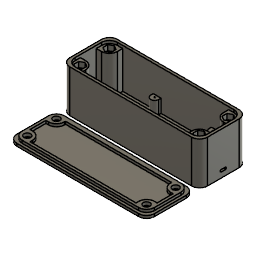
RGB Box v1 (Autodesk Fusion 360 design; units mm, degrees)
Autodesk Fusion 360 part; units mm, degrees
sketch "Sketch1" plane through (0, 0, 0) normal (0, 1, 0) x (1, 0, 0)
  line L0 (0, 0) -> (127, 0)
  line L1 (127, 0) -> (127, 40.64)
  line L2 (127, 40.64) -> (0, 40.64)
  line L3 (0, 40.64) -> (0, 0)
  line L4 (-2.54, -2.54) -> (129.54, -2.54)
  line L5 (129.54, -2.54) -> (129.54, 43.18)
  line L6 (129.54, 43.18) -> (-2.54, 43.18)
  line L7 (-2.54, 43.18) -> (-2.54, -2.54)
  line L8 (129.54, -2.54) -> (110.49, -2.54)
  line L9 (110.49, -2.54) -> (110.49, 16.51)
  line L10 (110.49, 16.51) -> (129.54, 16.51)
  line L11 (129.54, 16.51) -> (129.54, -2.54)
  line L12 (129.54, 43.18) -> (110.49, 43.18)
  line L13 (110.49, 43.18) -> (110.49, 24.13)
  line L14 (110.49, 24.13) -> (129.54, 24.13)
  line L15 (129.54, 24.13) -> (129.54, 43.18)
  dimension "d1" = 127
  dimension "d2" = 40.64
  dimension "d3" = 2.54
  dimension "d45" = 19.05
  dimension "d46" = 19.05
  dimension "d47" = 19.05
  dimension "d48" = 19.05
  constraint horizontal L0
  constraint vertical L1
  constraint horizontal L2
  constraint vertical L3
  constraint coincident L0.start L3.end
  constraint horizontal L8
  constraint vertical L9
  constraint horizontal L10
  constraint vertical L11
  constraint horizontal L12
  constraint vertical L13
  constraint horizontal L14
  constraint vertical L15
  measures "d1" distance of L0.start L0.end
  measures "d2" distance of L0.start L2.end
  measures "d45" distance of L4.end L8.end
  measures "d46" distance of L4.end L10.end
  measures "d47" distance of L5.end L12.end
  measures "d48" distance of L5.end L14.end
extrude "Extrude1" add sketch "Sketch1" along normal blind 40.64 makes body 1
shell "Shell1" thickness 2.54 removed faces 1 at (72.8133, 40.64, -12.7) on bodies 1
fillet "Fillet1" radius 7.62 8 edges at (0, 21.59, -40.64) (-2.54, 20.32, -43.18) (0, 21.59, 0) (-2.54, 20.32, 2.54) (127, 21.59, -40.64) (129.54, 20.32, -43.18) (127, 21.59, 0) (129.54, 20.32, 2.54) on bodies 1
sketch "Sketch2" plane through (-2.54, 0, 0) normal (-1, 0, 0) x (0, 0, 1)
  line L0 (-5.08, 0) -> (-5.08, 40.64)
  line L1 (-5.08, 40.64) -> (-35.56, 40.64)
  line L2 (-35.56, 40.64) -> (-35.56, 0)
  line L3 (-35.56, 0) -> (-5.08, 0)
  line L4 (-20.32, 0) -> (-20.32, 2.54)
  line L5 (-20.32, 2.54) -> (-20.32, 3.429)
  circle A0 centre (-20.32, 8.3185) radius 4.8895
  circle A1 centre (-20.32, 8.3185) radius 3.4925
  line L6 (-25.2095, 8.3185) -> (-15.4305, 8.3185)
  line L7 (-15.4305, 8.3185) -> (-15.4305, 0)
  line L8 (-15.4305, 0) -> (-25.2095, 0)
  line L9 (-25.2095, 0) -> (-25.2095, 8.3185)
  line L10 (-15.4305, 0) -> (-14.1605, 0)
  line L11 (-14.1605, 0) -> (-14.1605, 8.3172)
  line L12 (-14.1605, 8.3172) -> (-15.4305, 8.3172)
  line L13 (-15.4305, 8.3172) -> (-15.4305, 0)
  line L14 (-25.2095, 8.3185) -> (-26.4795, 8.3185)
  line L15 (-26.4795, 8.3185) -> (-26.4795, 0)
  line L16 (-26.4795, 0) -> (-25.2095, 0)
  line L17 (-25.2095, 0) -> (-25.2095, 8.3185)
  dimension "d9" = 0.889
  dimension "d10" = 9.779
  dimension "d11" = 6.985
  dimension "d12" = 9.779
  dimension "d16" = 1.27
  dimension "d17" = 1.27
  constraint midpoint L3 L4.start
  constraint perpendicular L3 L4
  constraint perpendicular L3 L5
  constraint coincident L5.end A0
  constraint concentric A0 A1
  constraint horizontal L6
  constraint vertical L7
  constraint horizontal L8
  constraint vertical L9
  constraint coincident L3 L7.end
  constraint coincident A0 L6.start
  constraint horizontal L10
  constraint vertical L11
  constraint horizontal L12
  constraint vertical L13
  constraint horizontal L14
  constraint vertical L15
  constraint horizontal L16
  constraint vertical L17
  constraint coincident L3 L15.end
  measures "d9" distance of L4.end L5.end
  measures "d10" diameter of A0
  measures "d11" diameter of A1
  measures "d12" distance of L6.start L6.end
  measures "d16" distance of L7.end L10.end
  measures "d17" distance of L6.start L14.end
extrude "Extrude2" add sketch "Sketch2" against normal blind 8.89 from surface at -2.54 contours L3 L7 L10 L11 L12 L13 | L3 L4 L5 A0 L7 L8 L13 | L3 L4 L5 A0 L8 L9 L17 | L3 L9 L14 L15 L16 L17 bodies 1
extrude "Extrude3" cut sketch "Sketch2" against normal blind 8.89 contours A1 L6 | A1 L6 bodies 1
sketch "Sketch3" plane through (0, 2.54, 0) normal (0, 1, 0) x (-1, 0, 0)
  line L0 (-8.89, -14.1605) -> (0, -14.1605)
  line L1 (0, -14.1605) -> (0, -7.62)
  arc A0 (0, -7.62) -> (-7.62, 0) centre (-7.62, -7.62) ccw
  line L2 (-7.62, 0) -> (-119.38, 0)
  arc A1 (-119.38, 0) -> (-127, -7.62) centre (-119.38, -7.62) ccw
  line L3 (-127, -7.62) -> (-127, -33.02)
  arc A2 (-127, -33.02) -> (-119.38, -40.64) centre (-119.38, -33.02) ccw
  line L4 (-119.38, -40.64) -> (-7.62, -40.64)
  arc A3 (-7.62, -40.64) -> (0, -33.02) centre (-7.62, -33.02) ccw
  line L5 (0, -33.02) -> (0, -26.4795)
  line L6 (0, -26.4795) -> (-8.89, -26.4795)
  line L7 (-8.89, -26.4795) -> (-8.89, -14.1605)
  line L8 (0, -14.1605) -> (-33.528, -14.1605)
  line L9 (-33.528, -14.1605) -> (-33.528, -26.4795)
  line L10 (-33.528, -26.4795) -> (-37.846, -26.4795)
  line L11 (-37.846, -26.4795) -> (-37.846, -14.1605)
  line L12 (-37.846, -14.1605) -> (-33.528, -14.1605)
  line L13 (-33.528, -14.1605) -> (-33.528, -26.4795)
  dimension "d20" = 33.528
  dimension "d21" = 4.318
  constraint coincident L0.end L1.start
  constraint perpendicular L1 L8
  constraint perpendicular L6 L9
  constraint horizontal L10
  constraint vertical L11
  constraint horizontal L12
  constraint vertical L13
  measures "d20" distance of L0.end L8.end
  measures "d21" distance of L9.end L10.end
extrude "Extrude4" add sketch "Sketch3" along normal blind 1.905 contours L9 L10 L11 L12 L13 bodies 1
sketch "Sketch4" plane through (129.54, 0, 0) normal (1, 0, 0) x (0, 0, -1)
  line L0 (5.08, 40.64) -> (5.08, 0)
  line L1 (5.08, 0) -> (35.56, 0)
  line L2 (35.56, 0) -> (35.56, 40.64)
  line L3 (35.56, 40.64) -> (5.08, 40.64)
  line L4 (20.32, 0) -> (20.32, 2.54)
  line L5 (20.32, 2.54) -> (20.32, 5.08)
  line L6 (20.32, 5.08) -> (20.32, 7.112)
  line L7 (20.32, 7.112) -> (17.526, 7.112)
  line L8 (17.526, 7.112) -> (23.114, 7.112)
  line L9 (17.526, 7.112) -> (23.114, 7.112)
  line L10 (23.114, 7.112) -> (23.114, 5.08)
  line L11 (23.114, 5.08) -> (17.526, 5.08)
  line L12 (17.526, 5.08) -> (17.526, 7.112)
  circle A0 centre (20.32, 10.16) radius 6.35
  dimension "d24" = 2.54
  dimension "d25" = 2.032
  dimension "d26" = 2.794
  dimension "d27" = 5.588
  constraint midpoint L1 L4.start
  constraint perpendicular L1 L4
  constraint parallel L4 L5
  constraint parallel L5 L6
  constraint perpendicular L6 L7
  constraint parallel L7 L8
  constraint horizontal L9
  constraint vertical L10
  constraint horizontal L11
  constraint vertical L12
  measures "d24" distance of L4.start L4.end
  measures "d25" distance of L5.end L6.end
  measures "d26" distance of L6.end L7.end
  measures "d27" distance of L7.end L8.end
extrude "Extrude5" cut sketch "Sketch4" against normal blind 6.35 contours L6 L7 L8 L9 L11 L12 | L6 L8 L9 L10 L11 bodies 1
fillet "Fillet2" radius 0.635 4 edges at (128.27, 7.112, -17.526) (128.27, 5.08, -17.526) (128.27, 5.08, -23.114) (128.27, 7.112, -23.114) on bodies 1
sketch "Sketch5" plane through (0, 2.54, 0) normal (0, 1, 0) x (-1, 0, 0)
  line L0 (-33.528, -14.1605) -> (-33.528, -26.4795)
  line L1 (-33.528, -26.4795) -> (-37.846, -26.4795)
  line L2 (-37.846, -26.4795) -> (-37.846, -14.1605)
  line L3 (-37.846, -14.1605) -> (-33.528, -14.1605)
  line L4 (-8.89, -14.1605) -> (0, -14.1605)
  line L5 (0, -14.1605) -> (0, -7.62)
  arc A0 (0, -7.62) -> (-7.62, 0) centre (-7.62, -7.62) ccw
  line L6 (-7.62, 0) -> (-119.38, 0)
  arc A1 (-119.38, 0) -> (-127, -7.62) centre (-119.38, -7.62) ccw
  line L7 (-127, -7.62) -> (-127, -33.02)
  arc A2 (-127, -33.02) -> (-119.38, -40.64) centre (-119.38, -33.02) ccw
  line L8 (-119.38, -40.64) -> (-7.62, -40.64)
  arc A3 (-7.62, -40.64) -> (0, -33.02) centre (-7.62, -33.02) ccw
  line L9 (0, -33.02) -> (0, -26.4795)
  line L10 (0, -26.4795) -> (-8.89, -26.4795)
  line L11 (-8.89, -26.4795) -> (-8.89, -14.1605)
  line L12 (-101.6, -20.32) -> (-101.6, -1.27)
  line L13 (-101.6, -1.27) -> (-101.6, -39.37)
  circle A4 centre (-101.6, -38.354) radius 1.016
  circle A5 centre (-101.6, -2.286) radius 1.016
  line L14 (-102.616, -2.286) -> (-44.704, -2.286)
  circle A6 centre (-45.72, -2.286) radius 1.016
  circle A7 centre (-45.72, -38.354) radius 1.016
  circle A8 centre (-101.6, -2.286) radius 3.81
  line L15 (-105.41, -2.286) -> (-105.41, 0)
  line L16 (-97.79, -2.286) -> (-97.79, 0)
  line L17 (-73.66, -2.286) -> (-73.66, -5.08)
  line L18 (-101.6, -20.32) -> (-99.06, -20.32)
  line L19 (-97.79, 0) -> (-105.41, 0)
  circle A9 centre (-45.72, -2.286) radius 3.81
  line L20 (-49.53, -2.286) -> (-49.53, 0)
  line L21 (-41.91, -2.286) -> (-41.91, 0)
  circle A10 centre (-101.6, -38.354) radius 3.81
  line L22 (-97.79, -38.354) -> (-97.79, -40.64)
  line L23 (-105.41, -38.354) -> (-105.41, -40.64)
  line L24 (-41.91, -38.354) -> (-41.91, -40.64)
  circle A11 centre (-45.72, -38.354) radius 3.81
  line L25 (-49.53, -38.354) -> (-49.53, -40.64)
  line L26 (-49.53, 0) -> (-41.91, 0)
  line L27 (-41.91, 0) -> (-49.53, 0)
  line L28 (-41.91, -40.64) -> (-49.53, -40.64)
  line L29 (-105.41, -40.64) -> (-97.79, -40.64)
  line L30 (-97.79, -40.64) -> (-105.41, -40.64)
  line L31 (-49.53, -40.64) -> (-41.91, -40.64)
  circle A12 centre (-101.6, -2.286) radius 0.635
  circle A13 centre (-101.6, -38.354) radius 0.635
  circle A14 centre (-45.72, -38.354) radius 0.635
  circle A15 centre (-45.72, -2.286) radius 0.635
  dimension "d32" = 19.05
  dimension "d33" = 38.1
  dimension "d34" = 2.032
  dimension "d35" = 2.032
  dimension "d36" = 57.912
  dimension "d37" = 2.032
  dimension "d38" = 2.032
  dimension "d39" = 1.27
  dimension "d40" = 1.27
  dimension "d41" = 1.27
  dimension "d42" = 1.27
  constraint perpendicular L8 L12
  constraint perpendicular L8 L13
  constraint coincident L13.end A4
  constraint coincident L12.end A5
  constraint coincident A5 L14.start
  constraint perpendicular L13 L14
  constraint coincident L14.end A6
  constraint concentric A5 A8
  constraint coincident A8 L15.start
  constraint coincident L6 L15.end
  constraint perpendicular L6 L15
  constraint coincident A8 L16.start
  constraint coincident L14 L16.start
  constraint coincident L6 L16.end
  constraint tangent A8 L16
  constraint midpoint L14 L17.start
  constraint perpendicular L14 L17
  constraint perpendicular L12 L18
  constraint symmetric A8 L17 A9
  constraint symmetric L15.start L17 L21.start
  constraint symmetric L15.end L17 L21.end
  constraint symmetric L16.start L17 L20.start
  constraint symmetric L16.end L17 L20.end
  constraint symmetric A8 L18 A10
  constraint symmetric L15.start L18 L23.start
  constraint symmetric L15.end L18 L23.end
  constraint symmetric L16.start L18 L22.start
  constraint symmetric L16.end L18 L22.end
  constraint symmetric L18 A9 A11
  constraint symmetric L18 L20.start L25.start
  constraint symmetric L18 L20.end L25.end
  constraint symmetric L18 L21.start L24.start
  constraint symmetric L18 L21.end L24.end
  constraint concentric A5 A12
  constraint concentric A4 A13
  constraint concentric A11 A14
  constraint concentric A6 A15
  measures "d32" distance of L12.start L12.end
  measures "d33" distance of L12.end L13.end
  measures "d34" diameter of A4
  measures "d35" diameter of A5
  measures "d36" distance of L14.start L14.end
  measures "d37" diameter of A6
  measures "d38" diameter of A7
  measures "d39" diameter of A12
  measures "d40" diameter of A13
  measures "d41" diameter of A14
  measures "d42" diameter of A15
extrude "Extrude6" add sketch "Sketch5" along normal blind 12.7 contours L6 A9 L21 L26 L27 | L6 A9 L26 L27 | L8 L24 A11 L28 L31 | L6 A9 L20 L26 L27 | L8 A11 L28 L31 | L8 A11 L25 L28 L31 | L6 A8 L16 L19 | L12 L13 A5 L14 A8 | L6 L12 L13 A5 L14 A8 L19 | L12 L13 A5 L14 A12 | L12 L13 A5 L14 A12 | L8 A10 L22 L29 L30 | L6 A8 L15 L19 | L12 L13 A5 L14 A12 | L12 L13 A5 L14 A12 | L8 A10 L29 L30 | L8 A10 L23 L29 L30 | L13 A4 A13 | L13 A4 A13 | L14 A6 A15 | L14 A6 A15 | A7 picked at (-45.7453, -0.4243) picked at (-45.7453, -40.2157) picked at (-101.6, -40.2167) bodies 1
sketch "Sketch6" plane through (0, 2.54, 0) normal (0, 1, 0) x (-1, 0, 0)
  line L0 (-33.528, -14.1605) -> (-33.528, -26.4795)
  line L1 (-33.528, -26.4795) -> (-37.846, -26.4795)
  line L2 (-37.846, -26.4795) -> (-37.846, -14.1605)
  line L3 (-37.846, -14.1605) -> (-33.528, -14.1605)
  line L4 (-41.91, 0) -> (-41.91, -2.286)
  arc A0 (-49.53, -2.286) -> (-41.91, -2.286) centre (-45.72, -2.286) ccw
  line L5 (-49.53, -2.286) -> (-49.53, 0)
  line L6 (-49.53, 0) -> (-97.79, 0)
  line L7 (-97.79, 0) -> (-97.79, -2.286)
  arc A1 (-105.41, -2.286) -> (-97.79, -2.286) centre (-101.6, -2.286) ccw
  line L8 (-105.41, -2.286) -> (-105.41, 0)
  line L9 (-105.41, 0) -> (-119.38, 0)
  arc A2 (-119.38, 0) -> (-127, -7.62) centre (-119.38, -7.62) ccw
  line L10 (-127, -7.62) -> (-127, -33.02)
  arc A3 (-127, -33.02) -> (-119.38, -40.64) centre (-119.38, -33.02) ccw
  line L11 (-119.38, -40.64) -> (-105.41, -40.64)
  line L12 (-105.41, -40.64) -> (-105.41, -38.354)
  arc A4 (-97.79, -38.354) -> (-105.41, -38.354) centre (-101.6, -38.354) ccw
  line L13 (-97.79, -38.354) -> (-97.79, -40.64)
  line L14 (-97.79, -40.64) -> (-49.53, -40.64)
  line L15 (-49.53, -40.64) -> (-49.53, -38.354)
  arc A5 (-41.91, -38.3588) -> (-49.53, -38.354) centre (-45.72, -38.354) ccw
  line L16 (-41.91, -38.3588) -> (-41.91, -40.64)
  line L17 (-41.91, -40.64) -> (-7.62, -40.64)
  arc A6 (-7.62, -40.64) -> (0, -33.02) centre (-7.62, -33.02) ccw
  line L18 (0, -33.02) -> (0, -26.4795)
  line L19 (0, -26.4795) -> (-8.89, -26.4795)
  line L20 (-8.89, -26.4795) -> (-8.89, -14.1605)
  line L21 (-8.89, -14.1605) -> (0, -14.1605)
  line L22 (0, -14.1605) -> (0, -7.62)
  arc A7 (0, -7.62) -> (-7.62, 0) centre (-7.62, -7.62) ccw
  line L23 (-7.62, 0) -> (-41.91, 0)
  line L24 (-127, 0) -> (-114.3, 0)
  line L25 (-114.3, 0) -> (-114.3, -5.08)
  line L26 (-121.92, -12.7) -> (-127, -12.7)
  line L27 (-127, -12.7) -> (-127, 0)
  line L28 (-116.6495, -4.0403) -> (-120.65, -1.7306)
  line L29 (-120.65, -1.7306) -> (-124.6505, -4.0403)
  line L30 (-124.6505, -4.0403) -> (-124.6505, -8.6597)
  line L31 (-124.6505, -8.6597) -> (-120.65, -10.9694)
  line L32 (-120.65, -10.9694) -> (-116.6495, -8.6597)
  line L33 (-116.6495, -8.6597) -> (-116.6495, -4.0403)
  circle A8 centre (-120.65, -6.35) radius 3.175
  line L34 (-10.3505, -4.0403) -> (-10.3505, -8.6597)
  line L35 (-2.3495, -8.6597) -> (-2.3495, -4.0403)
  circle A9 centre (-6.35, -6.35) radius 3.175
  line L36 (0, -12.7) -> (-5.08, -12.7)
  line L37 (-10.3505, -8.6597) -> (-6.35, -10.9694)
  line L38 (-6.35, -1.7306) -> (-10.3505, -4.0403)
  line L39 (-2.3495, -4.0403) -> (-6.35, -1.7306)
  line L40 (-12.7, -5.08) -> (-12.7, 0)
  line L41 (-12.7, 0) -> (0, 0)
  line L42 (-6.35, -10.9694) -> (-2.3495, -8.6597)
  line L43 (0, 0) -> (0, -12.7)
  line L44 (-124.6505, -31.9803) -> (-124.6505, -36.5997)
  line L45 (-116.6495, -36.5997) -> (-116.6495, -31.9803)
  circle A10 centre (-120.65, -34.29) radius 3.175
  line L46 (-114.3, -40.64) -> (-127, -40.64)
  line L47 (-124.6505, -36.5997) -> (-120.65, -38.9094)
  line L48 (-120.65, -29.6706) -> (-124.6505, -31.9803)
  line L49 (-116.6495, -31.9803) -> (-120.65, -29.6706)
  line L50 (-127, -40.64) -> (-127, -27.94)
  line L51 (-127, -27.94) -> (-121.92, -27.94)
  line L52 (-120.65, -38.9094) -> (-116.6495, -36.5997)
  line L53 (-114.3, -35.56) -> (-114.3, -40.64)
  line L54 (-10.3505, -31.9803) -> (-10.3505, -36.5997)
  line L55 (-2.3495, -36.5997) -> (-2.3495, -31.9803)
  circle A11 centre (-6.35, -34.29) radius 3.175
  line L56 (0, -40.64) -> (-12.7, -40.64)
  line L57 (-10.3505, -36.5997) -> (-6.35, -38.9094)
  line L58 (-6.35, -29.6706) -> (-10.3505, -31.9803)
  line L59 (-2.3495, -31.9803) -> (-6.35, -29.6706)
  line L60 (-12.7, -40.64) -> (-12.7, -35.56)
  line L61 (-5.08, -27.94) -> (0, -27.94)
  line L62 (-6.35, -38.9094) -> (-2.3495, -36.5997)
  line L63 (0, -27.94) -> (0, -40.64)
  arc A12 (-121.92, -12.7) -> (-114.3, -5.08) centre (-121.92, -5.08) ccw
  arc A13 (-114.3, -35.56) -> (-121.92, -27.94) centre (-121.92, -35.56) ccw
  arc A14 (-5.08, -27.94) -> (-12.7, -35.56) centre (-5.08, -35.56) ccw
  arc A15 (-12.7, -5.08) -> (-5.08, -12.7) centre (-5.08, -5.08) ccw
  line L64 (-129.54, 2.54) -> (2.54, 2.54)
  line L65 (2.54, 2.54) -> (2.54, -43.18)
  line L66 (2.54, -43.18) -> (-129.54, -43.18)
  line L67 (-129.54, -43.18) -> (-129.54, 2.54)
  line L68 (-114.3, 10.16) -> (-119.38, 10.16)
  line L69 (-124.6505, 14.2003) -> (-120.65, 11.8906)
  line L70 (-129.54, 15.24) -> (-129.54, 45.72)
  line L71 (-127, 38.1) -> (-127, 43.18)
  line L72 (-114.3, 15.24) -> (-114.3, 10.16)
  line L73 (-127, 17.78) -> (-127, 22.86)
  circle A16 centre (-120.65, 44.45) radius 3.175
  line L74 (-5.08, 7.62) -> (-121.92, 7.62)
  line L75 (-120.65, 49.0694) -> (-124.6505, 46.7597)
  line L76 (-121.92, 38.1) -> (-127, 38.1)
  line L77 (-114.3, 50.8) -> (-114.3, 45.72)
  line L78 (-119.38, 50.8) -> (-114.3, 50.8)
  line L79 (-127, 22.86) -> (-121.92, 22.86)
  line L80 (-124.6505, 42.1403) -> (-120.65, 39.8306)
  line L81 (-2.3495, 46.7597) -> (-6.35, 49.0694)
  line L82 (-2.3495, 42.1403) -> (-2.3495, 46.7597)
  line L83 (-10.3505, 14.2003) -> (-6.35, 11.8906)
  line L84 (0, 22.86) -> (0, 17.78)
  line L85 (-6.35, 39.8306) -> (-2.3495, 42.1403)
  line L86 (-2.3495, 18.8197) -> (-6.35, 21.1294)
  line L87 (-116.6495, 14.2003) -> (-116.6495, 18.8197)
  line L88 (-124.6505, 46.7597) -> (-124.6505, 42.1403)
  line L89 (-121.92, 53.34) -> (-5.08, 53.34)
  line L90 (2.54, 45.72) -> (2.54, 15.24)
  line L91 (-116.6495, 46.7597) -> (-120.65, 49.0694)
  line L92 (-120.65, 11.8906) -> (-116.6495, 14.2003)
  line L93 (0, 43.18) -> (0, 38.1)
  arc A17 (-12.7, 45.72) -> (-5.08, 38.1) centre (-5.08, 45.72) ccw
  line L94 (-12.7, 10.16) -> (-12.7, 15.24)
  circle A18 centre (-120.65, 16.51) radius 3.175
  line L95 (-7.62, 10.16) -> (-12.7, 10.16)
  line L96 (-124.6505, 18.8197) -> (-124.6505, 14.2003)
  line L97 (-116.6495, 18.8197) -> (-120.65, 21.1294)
  line L98 (-116.6495, 42.1403) -> (-116.6495, 46.7597)
  line L99 (-12.7, 50.8) -> (-7.62, 50.8)
  line L100 (-6.35, 21.1294) -> (-10.3505, 18.8197)
  line L101 (-6.35, 49.0694) -> (-10.3505, 46.7597)
  line L102 (-10.3505, 42.1403) -> (-6.35, 39.8306)
  line L103 (-6.35, 11.8906) -> (-2.3495, 14.2003)
  circle A19 centre (-6.35, 16.51) radius 3.175
  circle A20 centre (-6.35, 44.45) radius 3.175
  line L104 (-5.08, 22.86) -> (0, 22.86)
  line L105 (-10.3505, 46.7597) -> (-10.3505, 42.1403)
  line L106 (-10.3505, 18.8197) -> (-10.3505, 14.2003)
  arc A21 (-5.08, 22.86) -> (-12.7, 15.24) centre (-5.08, 15.24) ccw
  line L107 (-2.3495, 14.2003) -> (-2.3495, 18.8197)
  line L108 (0, 38.1) -> (-5.08, 38.1)
  line L109 (-120.65, 39.8306) -> (-116.6495, 42.1403)
  line L110 (-12.7, 45.72) -> (-12.7, 50.8)
  arc A22 (-121.92, 38.1) -> (-114.3, 45.72) centre (-121.92, 45.72) ccw
  arc A23 (-114.3, 15.24) -> (-121.92, 22.86) centre (-121.92, 15.24) ccw
  line L111 (-120.65, 21.1294) -> (-124.6505, 18.8197)
  arc A24 (-129.54, 15.24) -> (-121.92, 7.62) centre (-121.92, 15.24) ccw
  arc A25 (-121.92, 53.34) -> (-129.54, 45.72) centre (-121.92, 45.72) ccw
  arc A26 (2.54, 45.72) -> (-5.08, 53.34) centre (-5.08, 45.72) ccw
  arc A27 (-5.08, 7.62) -> (2.54, 15.24) centre (-5.08, 15.24) ccw
  arc A28 (-119.38, 50.8) -> (-127, 43.18) centre (-119.38, 43.18) ccw
  arc A29 (-127, 17.78) -> (-119.38, 10.16) centre (-119.38, 17.78) ccw
  arc A30 (-7.62, 10.16) -> (0, 17.78) centre (-7.62, 17.78) ccw
  arc A31 (0, 43.18) -> (-7.62, 50.8) centre (-7.62, 43.18) ccw
  line L112 (-127, 38.1) -> (-124.46, 38.1)
  line L113 (-124.46, 38.1) -> (-124.46, 22.86)
  line L114 (-124.46, 22.86) -> (-127, 22.86)
  line L115 (-127, 22.86) -> (-127, 38.1)
  line L116 (-114.3, 10.16) -> (-12.7, 10.16)
  line L117 (-12.7, 10.16) -> (-12.7, 14.2003)
  line L118 (-12.7, 14.2003) -> (-114.3, 14.2003)
  line L119 (-114.3, 14.2003) -> (-114.3, 10.16)
  line L120 (0, 22.86) -> (-2.54, 22.86)
  line L121 (-2.54, 22.86) -> (-2.54, 38.1)
  line L122 (-2.54, 38.1) -> (0, 38.1)
  line L123 (0, 38.1) -> (0, 22.86)
  line L124 (-12.7, 50.8) -> (-114.3, 50.8)
  line L125 (-114.3, 50.8) -> (-114.3, 48.26)
  line L126 (-114.3, 48.26) -> (-12.7, 48.26)
  line L127 (-12.7, 48.26) -> (-12.7, 50.8)
  circle A32 centre (-6.35, 44.45) radius 5
  circle A33 centre (-6.35, 16.51) radius 5
  circle A34 centre (-120.65, 16.51) radius 5
  circle A35 centre (-120.65, 44.45) radius 5
  point P0 (-120.65, -6.35)
  point P1 (-6.35, -6.35)
  point P2 (-120.65, -34.29)
  point P3 (-6.35, -34.29)
  point P4 (-6.35, 44.45)
  point P5 (-120.65, 16.51)
  point P6 (-6.35, 16.51)
  point P7 (-120.65, 44.45)
  dimension "d49" = 4.0005
  dimension "d50" = 6.35
  dimension "d55" = 7.62
  dimension "d56" = 7.62
  dimension "d57" = 7.62
  dimension "d58" = 7.62
  dimension "d67" = 4.0005
  dimension "d68" = 6.35
  dimension "d69" = 7.62
  dimension "d70" = 7.62
  dimension "d71" = 7.62
  dimension "d72" = 7.62
  dimension "d73" = 7.62
  dimension "d74" = 7.62
  dimension "d75" = 7.62
  dimension "d76" = 7.62
  dimension "d77" = 7.62
  dimension "d78" = 7.62
  dimension "d79" = 7.62
  dimension "d80" = 7.62
  dimension "d83" = 10
  dimension "d84" = 10
  dimension "d85" = 10
  dimension "d86" = 10
  constraint horizontal L24
  constraint vertical L25
  constraint horizontal L26
  constraint vertical L27
  constraint coincident P0 A8.centre
  constraint tangent L26 A12
  constraint tangent L25 A12
  constraint tangent L51 A13
  constraint tangent L53 A13
  constraint tangent L61 A14
  constraint tangent L60 A14
  constraint tangent L40 A15
  constraint tangent L36 A15
  constraint horizontal L64
  constraint vertical L65
  constraint horizontal L66
  constraint vertical L67
  constraint horizontal L78
  constraint vertical L77
  constraint horizontal L76
  constraint vertical L71
  constraint coincident P7 A16.centre
  constraint tangent L76 A22
  constraint tangent L77 A22
  constraint tangent L79 A23
  constraint tangent L72 A23
  constraint tangent L104 A21
  constraint tangent L94 A21
  constraint tangent A17 L110
  constraint tangent A17 L108
  constraint horizontal L89
  constraint vertical L90
  constraint horizontal L74
  constraint vertical L70
  constraint tangent L70 A24
  constraint tangent L74 A24
  constraint tangent L89 A25
  constraint tangent L70 A25
  constraint tangent L89 A26
  constraint tangent L90 A26
  constraint tangent L90 A27
  constraint tangent L74 A27
  constraint tangent L78 A28
  constraint tangent L71 A28
  constraint tangent L73 A29
  constraint tangent L68 A29
  constraint tangent L84 A30
  constraint tangent L95 A30
  constraint tangent L99 A31
  constraint tangent L93 A31
  constraint horizontal L112
  constraint vertical L113
  constraint horizontal L114
  constraint vertical L115
  constraint midpoint L79 L113.end
  constraint horizontal L116
  constraint vertical L117
  constraint horizontal L118
  constraint vertical L119
  constraint coincident L94 L117.end
  constraint horizontal L120
  constraint vertical L121
  constraint horizontal L122
  constraint vertical L123
  constraint midpoint L108 L121.end
  constraint horizontal L124
  constraint vertical L125
  constraint horizontal L126
  constraint vertical L127
  constraint midpoint L77 L125.end
  constraint concentric A20 A32
  constraint concentric A19 A33
  constraint concentric A18 A34
  measures "d49" distance of P0 L33
  measures "d50" diameter of A8
  measures "d55" radius of A12
  measures "d56" radius of A13
  measures "d57" radius of A14
  measures "d58" radius of A15
  measures "d67" distance of P7 L98
  measures "d68" diameter of A16
  measures "d69" radius of A22
  measures "d70" radius of A23
  measures "d71" radius of A21
  measures "d72" radius of A17
  measures "d73" radius of A24
  measures "d74" radius of A25
  measures "d75" radius of A26
  measures "d76" radius of A27
  measures "d77" radius of A28
  measures "d78" radius of A29
  measures "d79" radius of A30
  measures "d80" radius of A31
  measures "d83" diameter of A32
  measures "d84" diameter of A33
  measures "d85" diameter of A34
  measures "d86" diameter of A35
extrude "Extrude7" add sketch "Sketch6" along normal blind 38.1 contours L22 A7 L23 L36 L40 L41 L43 A15 | L9 A2 L10 L24 L25 L26 L27 A12 | L17 A6 L18 L56 L60 L61 L63 A14 | L10 A3 L11 L46 L50 L51 L53 A13 bodies 1
extrude "Extrude8" add sketch "Sketch6" along normal blind 30.48 contours L28 L29 L30 L31 L32 L33 | L34 L35 L37 L38 L39 L42 | L44 L45 L47 L48 L49 L52 | L54 L55 L57 L58 L59 L62 bodies 1
extrude "Extrude9" add 1 faces at (2.9633, 4.4657, -14.1605) along direction (0, 0, 1) blind 7.62 on bodies 1 bodies 1
extrude "Extrude10" add 1 faces at (2.9633, 6.3923, -26.4795) along direction (0, 0, -1) blind 6.35 on bodies 1 bodies 1
extrude "Extrude11" add sketch "Sketch6" along normal blind 2.54 separate body contours L68 L72 L73 L79 A23 A29 L114 L119 | L72 L94 L116 L117 L118 L119 | L72 L76 L77 L79 A17 L94 L104 A21 L108 L110 A22 A23 L113 L118 L121 L126 | L84 L94 L95 L104 A21 A30 L117 L120 | L76 L79 L112 L113 L114 L115 | L71 L76 L77 L78 A22 A28 L112 L125 | L104 L108 L120 L121 L122 L123 | L93 A17 L99 L108 L110 A31 L122 L127 | L77 L110 L124 L125 L126 L127 | L69 L87 L92 L96 L97 L111 | L70 L74 L89 L90 A24 A25 A26 A27 | L75 L80 L88 L91 L98 L109 | L81 L82 L85 L101 L102 L105 | L83 L86 L100 L103 L106 L107 | A32 | A33 | A34 | A35 makes body 2
extrude "Extrude12" add sketch "Sketch6" along normal blind 5.08 contours L68 L72 L73 L79 A23 A29 L114 L119 | L72 L94 L116 L117 L118 L119 | L84 L94 L95 L104 A21 A30 L117 L120 | L76 L79 L112 L113 L114 L115 | L71 L76 L77 L78 A22 A28 L112 L125 | L104 L108 L120 L121 L122 L123 | L93 A17 L99 L108 L110 A31 L122 L127 | L77 L110 L124 L125 L126 L127 | L69 L87 L92 L96 L97 L111 | L75 L80 L88 L91 L98 L109 | L81 L82 L85 L101 L102 L105 | L83 L86 L100 L103 L106 L107 | A32 | A33 | A34 | A35 bodies 2
extrude "Extrude13" cut sketch "Sketch6" along normal blind 2 contours L69 L87 L92 L96 L97 L111 | A16 | L75 L80 L88 L91 L98 L109 | L81 L82 L85 L101 L102 L105 | L83 L86 L100 L103 L106 L107 | A18 | A19 | A20 | A32 | A33 | A34 | A35 bodies 2
extrude "Extrude14" [suppressed]
move_body "Move1" bodies 2 to x (1, 0, 0) y (0, 1, 0) z (0, 0, 1) at (0, -2.54, 0)
extrude "Extrude15" cut sketch "Sketch6" against normal blind 2.54 from surface at 38.1 contours L22 A7 L23 L36 L40 L41 L43 A15 | L9 A2 L10 L24 L25 L26 L27 A12 | L17 A6 L18 L56 L60 L61 L63 A14 | L10 A3 L11 L46 L50 L51 L53 A13 bodies 1
equation "d26 = ( 0.22 / 2 ) * 1 in"
equation "d49 = ( 0.315 / 2 ) * 1 in"
equation "d67 = ( 0.315 / 2 ) * 1 in"
